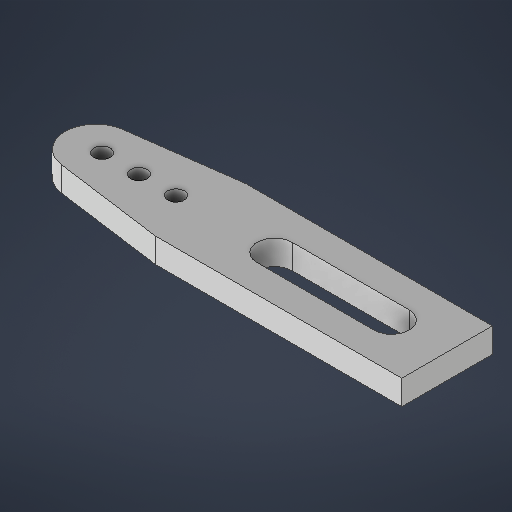
# Autodesk Inventor part: MMAE 232 CAD Assignment 2 Servo Horn 1-Nicholas Skiba
Saved by Autodesk Inventor 2026.1 (Build 301233000, 233)
## iProperties
Created: 2025-08-27
Part Number: MMAE 232 CAD Assignment 2 Servo Horn 1-Nicholas Skiba
Material: Generic
Document SubType Name: Modeling
Designer: Nick
Density: 1 g/cm^3
Appearance: Default
Author: Nick
Autodesk Inventor part; units mm, degrees
ref_plane "YZ Plane" through (0, 0, 0) normal (1, 0, 0) x (0, 1, 0)
ref_plane "XZ Plane" through (0, 0, 0) normal (0, 1, 0) x (-1, 0, 0)
ref_plane "XY Plane" through (0, 0, 0) normal (0, 0, 1) x (1, 0, 0)
sketch "Sketch1" plane through (0, 0, 0) normal (0, 1, 0) x (-1, 0, 0)
  line L0 (0, 0) -> (0, -7.35)
  line L1 (0, -7.35) -> (20, -7.35)
  line L2 (0, 0) -> (20, 0)
  line L3 (0, 0) -> (0, -3.68)
  line L4 (0, -3.68) -> (4.5, -3.68) construction
  line L5 (4.5, -3.68) -> (14, -3.68) construction
  line L6 (14, -3.68) -> (22, -3.68) construction
  line L7 (22, -3.68) -> (25, -3.68) construction
  line L8 (25, -3.68) -> (28, -3.68) construction
  line L9 (28, -3.68) -> (28.5, -3.68) construction
  arc A0 (28.8344, -6.1575) -> (28.8372, -1.2028) centre (28.5, -3.68) ccw
  circle A1 centre (28, -3.68) radius 0.67
  circle A2 centre (25, -3.68) radius 0.67
  circle A3 centre (22, -3.68) radius 0.67
  line L10 (20, 0) -> (28.8372, -1.2028)
  line L11 (20, -7.35) -> (28.8344, -6.1575)
  arc A4 (4.5, -2.255) -> (4.5, -5.105) centre (4.5, -3.68) ccw
  arc A5 (14, -5.105) -> (14, -2.255) centre (14, -3.68) ccw
  line L12 (14, -2.255) -> (4.5, -2.255)
  line L13 (4.5, -5.105) -> (14, -5.105)
  dimension "d0" = 7.35
  dimension "d1" = 20
  dimension "d2" = 20
  dimension "d3" = 3.68
  dimension "d4" = 4.5
  dimension "d5" = 9.5
  dimension "d6" = 8
  dimension "d7" = 3
  dimension "d8" = 3
  dimension "d9" = 0.5
  dimension "d10" = 5
  dimension "d11" = 1.34
  dimension "d12" = 1.34
  dimension "d13" = 1.34
  dimension "d16" = 2.85
  dimension "d17" = 2.85
  constraints: 28 end point, 6 centre point, 6 coincident, 6 point on circle, 6 point on line, 5 tangent, 2 horizontal, 2 perpendicular, 1 vertical
  measures "d0" distance of L0.start L0.end
  measures "d1" distance of L0.end L1.end
  measures "d2" distance of L0.start L2.end
  measures "d3" distance of L0.start L3.end
  measures "d4" distance of L3.end L4.end
  measures "d5" distance of L4.end L5.end
  measures "d6" distance of L5.end L6.end
  measures "d7" distance of L6.end L7.end
  measures "d8" distance of L7.end L8.end
  measures "d9" distance of L8.end L9.end
  measures "d10" diameter of A0
  measures "d11" diameter of A1
  measures "d12" diameter of A2
  measures "d13" diameter of A3
  measures "d16" diameter of A4
  measures "d17" diameter of A5
extrude "Extrusion1" add sketch "Sketch1" along normal blind 2
body "Solid1"
